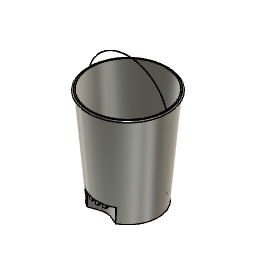
BALDE v2 (Autodesk Fusion 360 design; units mm, degrees)
Autodesk Fusion 360 part; units mm, degrees
note: some values were not read from the file. Set by a fixed rule: which sketch regions a step uses.
sketch "Sketch1" plane through (0, 0, 0) normal (0, 0, 1) x (1, 0, 0)
  circle A0 centre (0, 0) radius 50
  dimension "d1" = 100
  constraint coincident A0.centre origin
  measures "d1" diameter of A0
extrude "Extrude1" add sketch "Sketch1" along normal blind 159 draft 5 makes body 1
sketch "Sketch2" plane through (0, 0, 159) normal (0, 0, 1) x (-1, 0, 0)
  circle A0 centre (0, 0) radius 63.9107
  circle A1 centre (0, 0) radius 66.5
  dimension "d4" = 133
  constraint coincident A0.centre A1.centre
  measures "d4" diameter of A1
extrude "Extrude2" add sketch "Sketch2" along normal blind 2 contours A0 | A1 bodies 1
fillet "Fillet1" radius 2 1 edges at (61.9998, 24.0474, 161) on bodies 1
sketch "Sketch3" plane through (0, 0, 0) normal (0, 0, -1) x (1, 0, 0)
  circle A0 centre (0, 0) radius 50
  spline S0 degree 2 poles (-23.3209, -44.2282) (-0.4593, -34.0196) (24.4337, -43.6233) knots 0 0 0 5.002367 5.002367 5.002367 weights 1 3 1
  spline S1 degree 2 poles (23.3209, 44.2282) (0.4593, 34.0196) (-24.4337, 43.6233) knots 0 0 0 5.002367 5.002367 5.002367 weights 1 3 1
  line L0 (-24.4337, 43.6233) -> (-65.2127, 59.3558)
  line L1 (-65.2127, 59.3558) -> (25.469, 113.112)
  line L2 (25.469, 113.112) -> (64.1313, 59.3558)
  line L3 (64.1313, 59.3558) -> (23.3209, 44.2282)
  line L4 (24.4337, -43.6233) -> (80.8509, -65.389)
  line L5 (80.8509, -65.389) -> (-53.5394, -115.2046)
  line L6 (-53.5394, -115.2046) -> (-62.5952, -59.3342)
  line L7 (-62.5952, -59.3342) -> (-23.3209, -44.2282)
  dimension "d10" = 360
  constraint coincident A0 S0.end
  constraint coincident A0 S0.start
  constraint parallel L3 L5
extrude "Extrude3" cut sketch "Sketch3" against normal blind 25 contours A0 S1 | A0 L0 L1 L2 L3 | A0 L4 L5 L6 L7 | A0 S0 bodies 1
sketch "Sketch4" plane through (0, 0, 25) normal (0, 0, -1) x (1, 0, 0)
  arc A0 (-25.9903, -45.2549) -> (27.0469, -44.6315) centre (0, 0) ccw
  line L0 (27.0469, -44.6315) -> (24.4337, -43.6233)
  spline S0 degree 2 poles (-23.3209, -44.2282) (-0.4593, -34.0196) (24.4337, -43.6233) knots 0 0 0 5.002367 5.002367 5.002367 weights 1 3 1
  line L1 (-23.3209, -44.2282) -> (-25.9903, -45.2549)
  line L2 (-2.5658, -36.6705) -> (2.5587, -36.6705)
  line L3 (2.5587, -36.6705) -> (2.5587, -52.1245)
  line L4 (2.5587, -52.1245) -> (-2.5658, -52.1245)
  line L5 (-2.5658, -52.1245) -> (-2.5658, -36.6705)
  line L6 (13.5587, -36.6705) -> (13.5587, -52.1245)
  line L7 (13.5587, -52.1245) -> (8.4342, -52.1245)
  line L8 (8.4342, -52.1245) -> (8.4342, -36.6705)
  line L9 (8.4342, -36.6705) -> (13.5587, -36.6705)
  line L10 (-13.5658, -52.1245) -> (-13.5658, -36.6705)
  line L11 (-13.5658, -36.6705) -> (-8.4413, -36.6705)
  line L12 (-8.4413, -36.6705) -> (-8.4413, -52.1245)
  line L13 (-8.4413, -52.1245) -> (-13.5658, -52.1245)
  line L14 (-2.5658, 36.8755) -> (-2.5658, 52.1128)
  line L15 (2.5587, 52.1128) -> (2.5587, 36.8755)
  line L16 (2.5587, 36.8755) -> (-2.5658, 36.8755)
  line L17 (13.5587, 50.41) -> (13.5587, 36.8755)
  line L18 (13.5587, 36.8755) -> (8.4342, 36.8755)
  line L19 (8.4342, 36.8755) -> (8.4342, 51.4967)
  line L20 (-13.5658, 36.8755) -> (-13.5658, 50.3884)
  line L21 (-8.4413, 36.8755) -> (-13.5658, 36.8755)
  line L22 (-8.4413, 51.4788) -> (-8.4413, 36.8755)
  spline S1 degree 2 poles (-8.4413, 51.4788) (-11.1565, 50.9881) (-13.5658, 50.3884) knots 0 0 0 0.524085 0.524085 0.524085 weights 1 3 1
  spline S2 degree 2 poles (-2.5658, 52.1128) (-0.0091, 52.2026) (2.5587, 52.1128) knots 0 0 0 0.512632 0.512632 0.512632 weights 1 3 1
  spline S3 degree 2 poles (8.4342, 51.4967) (10.9338, 51.0429) (13.5587, 50.41) knots 0 0 0 0.52397 0.52397 0.52397 weights 1 3 1
  constraint horizontal L2
  constraint vertical L3
  constraint horizontal L4
  constraint vertical L5
  constraint coincident A0 L3.end
  constraint coincident S0 L2.start
  constraint horizontal L9
  constraint vertical L6
  constraint horizontal L7
  constraint vertical L8
  constraint horizontal L11
  constraint vertical L12
  constraint horizontal L13
  constraint vertical L10
  constraint vertical L15
  constraint horizontal L16
  constraint vertical L14
  constraint vertical L17
  constraint horizontal L18
  constraint vertical L19
  constraint vertical L22
  constraint horizontal L21
  constraint vertical L20
extrude "Extrude4" add sketch "Sketch4" along normal blind 5 contours L2 L3 L4 L5 | A0 S0 L10 L12 | A0 S0 L6 L8 | L14 L15 L16 S2 | L17 L18 L19 S3 | L20 L21 L22 S1 bodies 1
sketch "Sketch5" plane through (0, 0, 161) normal (0, 0, 1) x (-1, 0, 0)
  circle A0 centre (0, 0) radius 64.5
  circle A1 centre (0, 0) radius 62.5
  dimension "d15" = 125
  constraint coincident A0.centre A1.centre
  measures "d15" diameter of A1
extrude "Extrude5" cut sketch "Sketch5" against normal blind 135 draft -5 contours A1 bodies 1
sketch "Sketch6" plane through (0, 0, 0) normal (0, 1, 0) x (1, 0, 0)
  arc A0 (-64.3402, -161.072) -> (64.4311, -161.1311) centre (0.0542, -142.058) ccw
  arc A1 (-64.1572, -161.072) -> (64.0079, -161.1311) centre (-0.0658, -141.8579) ccw
  line L0 (64.4311, -161.1311) -> (64.0079, -161.1311)
  line L1 (-64.1572, -161.072) -> (-64.3402, -161.072)
  constraint tangent A0 A1
  constraint horizontal L0
  constraint parallel L0 L1
extrude "Extrude6" add sketch "Sketch6" along normal blind 0.1 separate body makes body 2
